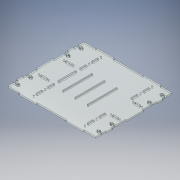
# Autodesk Inventor part: Base
Saved by Autodesk Inventor 2019 (Build 230136000, 136)
## iProperties
Created: 2020-04-02
Part Number: Base
Material: Acetal Resin, White
Document SubType Name: Modeling
Designer: Jurgen
Density: 1.425 g/cm^3
Appearance: Clear
Author: Jurgen
Autodesk Inventor part; units mm, degrees
(part 1 of 2)
ref_plane "YZ Plane" through (0, 0, 0) normal (1, 0, 0) x (0, 1, 0)
ref_plane "XZ Plane" through (0, 0, 0) normal (0, 1, 0) x (-1, 0, 0)
ref_plane "XY Plane" through (0, 0, 0) normal (0, 0, 1) x (1, 0, 0)
sketch "Sketch1" plane through (0, 0, 0) normal (0, 1, 0) x (-1, 0, 0)
  line L0 (-230, -200) -> (50, -200)
  line L1 (50, -200) -> (50, 60)
  line L2 (50, 60) -> (-230, 60)
  line L3 (-230, 60) -> (-230, -200)
  line L4 (-230, -200) -> (50, 60) construction
  line L5 (50, -200) -> (-230, 60) construction
  line L6 (0, 60) -> (0, -200) construction
  line L7 (-170, 60) -> (-170, -200) construction
  line L8 (50, -70) -> (-230, -70) construction
  line L9 (-90, 60) -> (-90, -200) construction
  dimension "d7" = 280
  dimension "d8" = 260
  dimension "d11" = 170
  dimension "d12" = 50
  constraints: 20 end point, 4 midpoint, 4 point on line, 2 horizontal, 2 parallel, 2 perpendicular, 1 vertical
  measures "d7" distance of L2.end L1.end
  measures "d8" distance of L1.end L0.end
  measures "d11" distance between parallel lines of L7 L6
  measures "d12" distance between parallel lines of L1 L6
extrude "Extrusion2" add sketch "Sketch1" along normal blind 5
sketch "Sketch2" plane through (0, 5, 0) normal (0, 1, 0) x (1, 0, 0)
  line L0 (230, 200) -> (-50, 200) construction
  line L1 (-50, 200) -> (-50, -60) construction
  line L2 (-50, -60) -> (230, -60) construction
  line L3 (230, -60) -> (230, 200) construction
  line L4 (-50, -60) -> (230, -60) construction
  line L5 (0, -60) -> (0, 200) construction
  line L6 (180, -60) -> (180, 200) construction
  line L7 (0, -35) -> (5, -35)
  line L8 (5, -35) -> (5, 25)
  line L9 (5, 25) -> (0, 25)
  line L10 (0, 25) -> (0, -35)
  line L11 (0, 115) -> (5, 115)
  line L12 (5, 115) -> (5, 175)
  line L13 (5, 175) -> (0, 175)
  line L14 (0, 175) -> (0, 115)
  line L15 (180, -35) -> (175, -35)
  line L16 (175, -35) -> (175, 25)
  line L17 (175, 25) -> (180, 25)
  line L18 (180, 25) -> (180, -35)
  line L19 (180, 115) -> (175, 115)
  line L20 (175, 115) -> (175, 175)
  line L21 (175, 175) -> (180, 175)
  line L22 (180, 175) -> (180, 115)
  point P0 (0, 0)
  dimension "d24" = 180
  dimension "d25" = 50
  dimension "d26" = 5
  dimension "d27" = 60
  dimension "d28" = 25
  dimension "d29" = 5
  dimension "d30" = 60
  dimension "d31" = 25
  dimension "d32" = 5
  dimension "d33" = 60
  dimension "d34" = 5
  dimension "d35" = 60
  dimension "d36" = 25
  dimension "d37" = 25
  constraints: 36 end point, 8 parallel, 8 point on line, 6 perpendicular, 4 horizontal
  measures "d24" distance between parallel lines of L6 L5
  measures "d25" distance between parallel lines of L1 L5
  measures "d26" distance of L9.end L8.end
  measures "d27" distance of L8.end L7.end
  measures "d28" distance between parallel lines of L2 L7
  measures "d29" distance of L13.end L12.end
  measures "d30" distance of L12.end L11.end
  measures "d31" distance between parallel lines of L0 L13
  measures "d32" distance of L16.end L17.end
  measures "d33" distance of L15.end L16.end
  measures "d34" distance of L20.end L21.end
  measures "d35" distance of L19.end L20.end
  measures "d36" distance from line of L2 L15.end
  measures "d37" distance from line of L6.end L21
extrude "Extrusion3" cut sketch "Sketch2" against normal blind 5
sketch "Sketch3" plane through (0, 5, 0) normal (0, 1, 0) x (1, 0, 0)
  line L0 (180, 25) -> (180, -35) construction
  line L1 (180, -35) -> (175, -35) construction
  line L2 (175, -35) -> (175, 25) construction
  line L3 (175, 25) -> (180, 25) construction
  line L4 (5, 25) -> (5, -35) construction
  line L5 (5, -35) -> (0, -35) construction
  line L6 (0, -35) -> (0, 25) construction
  line L7 (0, 25) -> (5, 25) construction
  line L8 (5, 175) -> (5, 115) construction
  line L9 (5, 115) -> (0, 115) construction
  line L10 (0, 115) -> (0, 175) construction
  line L11 (0, 175) -> (5, 175) construction
  line L12 (180, 175) -> (180, 115) construction
  line L13 (180, 115) -> (175, 115) construction
  line L14 (175, 115) -> (175, 175) construction
  line L15 (175, 175) -> (180, 175) construction
  line L16 (230, 200) -> (-50, 200) construction
  line L17 (-50, 200) -> (-50, -60) construction
  line L18 (-50, -60) -> (230, -60) construction
  line L19 (230, -60) -> (230, 200) construction
  line L20 (90, 200) -> (90, -60) construction
  line L21 (-50, -60) -> (230, -60) construction
  line L22 (-50, 200) -> (-50, -60) construction
  line L23 (-50, 70) -> (230, 70) construction
  line L24 (190, -60) -> (190, 200) construction
  line L25 (205, 30) -> (225, 30)
  line L26 (225, 30) -> (225, 25)
  line L27 (225, 25) -> (205, 25)
  line L28 (205, 25) -> (205, 30)
  line L29 (205, 110) -> (225, 110)
  line L30 (225, 110) -> (225, 115)
  line L31 (225, 115) -> (205, 115)
  line L32 (205, 115) -> (205, 110)
  line L33 (-25, 30) -> (-45, 30)
  line L34 (-45, 30) -> (-45, 25)
  line L35 (-45, 25) -> (-25, 25)
  line L36 (-25, 25) -> (-25, 30)
  line L37 (-45, 115) -> (-25, 115)
  line L38 (-45, 110) -> (-45, 115)
  line L39 (-25, 110) -> (-45, 110)
  line L40 (-25, 115) -> (-25, 110)
  point P0 (0, 0)
  dimension "d40" = 20
  dimension "d41" = 5
  dimension "d43" = 15
  dimension "d48" = 30
  dimension "d58" = 80
  constraints: 38 end point, 12 symmetric about line, 4 midpoint, 2 parallel, 2 perpendicular, 2 point on line, 1 horizontal
  measures "d40" distance of L26.end L27.end
  measures "d41" distance of L25.end L26.end
  measures "d43" distance between parallel lines of L24 L28
  measures "d48" distance from line of L29.start L14
  measures "d58" distance between parallel lines of L25 L29
extrude "Extrusion5" cut sketch "Sketch3" against normal blind 10 contours L36 L35 L34 L33 | L37 L40 L39 L38
sketch "Sketch6" plane through (0, 5, 0) normal (0, 1, 0) x (1, 0, 0)
  line L0 (-45, 115) -> (-25, 115) construction
  line L1 (-25, 115) -> (-25, 110) construction
  line L2 (-25, 110) -> (-45, 110) construction
  line L3 (-45, 30) -> (-25, 30) construction
  line L4 (-25, 30) -> (-25, 25) construction
  line L5 (-25, 25) -> (-45, 25) construction
  line L6 (180, 25) -> (180, -35) construction
  line L7 (180, -35) -> (175, -35) construction
  line L8 (175, -35) -> (175, 25) construction
  line L9 (175, 25) -> (180, 25) construction
  line L10 (5, 25) -> (5, -35) construction
  line L11 (5, -35) -> (0, -35) construction
  line L12 (0, -35) -> (0, 25) construction
  line L13 (0, 25) -> (5, 25) construction
  line L14 (5, 175) -> (5, 115) construction
  line L15 (5, 115) -> (0, 115) construction
  line L16 (0, 115) -> (0, 175) construction
  line L17 (0, 175) -> (5, 175) construction
  line L18 (180, 175) -> (180, 115) construction
  line L19 (180, 115) -> (175, 115) construction
  line L20 (175, 115) -> (175, 175) construction
  line L21 (175, 175) -> (180, 175) construction
  line L22 (230, 200) -> (-50, 200) construction
  line L23 (-50, 200) -> (-50, -60) construction
  line L24 (-50, -60) -> (230, -60) construction
  line L25 (230, -60) -> (230, 200) construction
  line L26 (230, 200) -> (-50, 200) projected
  line L27 (-50, -60) -> (230, -60) projected
  line L28 (230, 200) -> (210, 200)
  line L29 (210, 200) -> (210, -60)
  line L30 (210, -60) -> (230, -60)
  line L31 (230, -60) -> (230, 200)
  line L32 (-45, 110) -> (-45, 115) projected
  line L33 (-45, 25) -> (-45, 30) projected
  point P0 (0, 0)
  dimension "d51" = 20
  constraints: 8 end point, 2 parallel, 1 horizontal, 1 perpendicular, 1 point on line
  measures "d51" distance of L30.end L29.end
extrude "Extrusion7" cut sketch "Sketch6" against normal blind 10
sketch "Sketch7" plane through (0, 5, 0) normal (0, 1, 0) x (1, 0, 0)
  line L0 (210, -60) -> (210, 200) construction
  line L1 (210, 200) -> (-50, 200) construction
  line L2 (-50, 200) -> (-50, -60) construction
  line L3 (-50, -60) -> (210, -60) construction
  line L4 (180, 175) -> (180, 115) construction
  line L5 (180, 115) -> (175, 115) construction
  line L6 (175, 115) -> (175, 175) construction
  line L7 (175, 175) -> (180, 175) construction
  line L8 (5, 175) -> (5, 115) construction
  line L9 (5, 115) -> (0, 115) construction
  line L10 (0, 115) -> (0, 175) construction
  line L11 (0, 175) -> (5, 175) construction
  line L12 (5, 25) -> (5, -35) construction
  line L13 (5, -35) -> (0, -35) construction
  line L14 (0, -35) -> (0, 25) construction
  line L15 (0, 25) -> (5, 25) construction
  line L16 (180, 25) -> (180, -35) construction
  line L17 (180, -35) -> (175, -35) construction
  line L18 (175, -35) -> (175, 25) construction
  line L19 (175, 25) -> (180, 25) construction
  line L20 (-45, 30) -> (-25, 30) construction
  line L21 (-25, 30) -> (-25, 25) construction
  line L22 (-25, 25) -> (-45, 25) construction
  line L23 (-45, 115) -> (-25, 115) construction
  line L24 (-25, 115) -> (-25, 110) construction
  line L25 (-25, 110) -> (-45, 110) construction
  line L26 (-50, 200) -> (-70, 200)
  line L27 (-70, 200) -> (-70, -60)
  line L28 (-70, -60) -> (-50, -60)
  line L29 (-50, -60) -> (-50, 200)
  line L30 (-45, 25) -> (-45, 30) projected
  line L31 (-45, 110) -> (-45, 115) projected
  point P0 (0, 0)
  dimension "d54" = 20
  dimension "d57" = 260
  constraints: 8 end point, 2 parallel, 1 horizontal, 1 perpendicular
  measures "d54" distance of L28.end L27.end
  measures "d57" distance of L26.end L27.end
extrude "Extrusion8" add sketch "Sketch7" against normal blind 5
sketch "Sketch8" plane through (210, 5, 60) normal (1, 0, 0) x (0, 0, -1)
  line L0 (260, -5) -> (0, -5) projected
  line L1 (260, 0) -> (260, -5) projected
  line L2 (0, 0) -> (260, 0) projected
  line L3 (0, -5) -> (0, 0) projected
  point P0 (60, -5)
extrude "Extrusion9" add sketch "Sketch8" along normal blind 20
sketch "Sketch9" plane through (0, 5, 0) normal (0, 1, 0) x (1, 0, 0)
  line L0 (230, 200) -> (-70, 200) construction
  line L1 (-70, 200) -> (-70, -60) construction
  line L2 (-70, -60) -> (230, -60) construction
  line L3 (230, 200) -> (230, -60) construction
  line L4 (180, 175) -> (180, 115) construction
  line L5 (180, 115) -> (175, 115) construction
  line L6 (175, 115) -> (175, 175) construction
  line L7 (175, 175) -> (180, 175) construction
  line L8 (5, 175) -> (5, 115) construction
  line L9 (5, 115) -> (0, 115) construction
  line L10 (0, 115) -> (0, 175) construction
  line L11 (0, 175) -> (5, 175) construction
  line L12 (5, 25) -> (5, -35) construction
  line L13 (5, -35) -> (0, -35) construction
  line L14 (0, -35) -> (0, 25) construction
  line L15 (0, 25) -> (5, 25) construction
  line L16 (180, 25) -> (180, -35) construction
  line L17 (180, -35) -> (175, -35) construction
  line L18 (175, -35) -> (175, 25) construction
  line L19 (175, 25) -> (180, 25) construction
  line L20 (-45, 30) -> (-25, 30) construction
  line L21 (-25, 30) -> (-25, 25) construction
  line L22 (-25, 25) -> (-45, 25) construction
  line L23 (-45, 115) -> (-25, 115) construction
  line L24 (-25, 115) -> (-25, 110) construction
  line L25 (-25, 110) -> (-45, 110) construction
  line L26 (5, 115) -> (5, 135) construction
  line L27 (5, 175) -> (5, 115) construction
  line L28 (0, 115) -> (0, 175) construction
  line L29 (5, 135) -> (0, 135)
  line L30 (0, 135) -> (0, 155)
  line L31 (0, 155) -> (5, 155)
  line L32 (5, 155) -> (5, 135)
  line L33 (2.5, 155) -> (2.5, 135) construction
  line L34 (0, 145) -> (5, 145) construction
  circle A0 centre (2.5, 145) radius 2
  line L35 (5, 115) -> (0, 115) construction
  line L36 (2.5, 115) -> (2.5, 200) construction
  line L37 (230, 200) -> (-70, 200) construction
  circle A1 centre (2.5, 185) radius 2
  line L38 (180, 135) -> (175, 135)
  line L39 (175, 135) -> (175, 155)
  line L40 (175, 155) -> (180, 155)
  line L41 (180, 155) -> (180, 135)
  line L42 (177.5, 155) -> (177.5, 135) construction
  line L43 (175, 145) -> (180, 145) construction
  circle A2 centre (177.5, 145) radius 2
  circle A3 centre (177.5, 185) radius 2
  line L44 (5, -15) -> (0, -15)
  line L45 (0, -15) -> (0, 5)
  line L46 (0, 5) -> (5, 5)
  line L47 (5, 5) -> (5, -15)
  line L48 (2.5, 5) -> (2.5, -15) construction
  line L49 (0, -5) -> (5, -5) construction
  circle A4 centre (2.5, -5) radius 2
  circle A5 centre (2.5, 35) radius 2
  line L50 (180, -15) -> (175, -15)
  line L51 (175, -15) -> (175, 5)
  line L52 (175, 5) -> (180, 5)
  line L53 (180, 5) -> (180, -15)
  line L54 (177.5, 5) -> (177.5, -15) construction
  line L55 (175, -5) -> (180, -5) construction
  circle A6 centre (177.5, -5) radius 2
  circle A7 centre (177.5, 35) radius 2
  line L56 (-45, 25) -> (-45, 30) projected
  line L57 (-45, 110) -> (-45, 115) projected
  point P0 (0, 0)
  dimension "d61" = 20
  dimension "d65" = 20
  dimension "d66" = 4
  dimension "d67" = 4
  dimension "d68" = 10
  dimension "d69" = 20
  dimension "d70" = 4
  dimension "d71" = 4
  dimension "d72" = 20
  dimension "d73" = 4
  dimension "d74" = 4
  dimension "d75" = 20
  dimension "d76" = 4
  dimension "d77" = 4
  constraints: 52 end point, 21 midpoint, 8 centre point, 8 parallel, 5 perpendicular, 4 horizontal, 4 point on line
  measures "d61" distance of L8.end L26.end
  measures "d65" distance of L29.end L30.end
  measures "d66" diameter of A0
  measures "d67" diameter of A1
  measures "d68" distance from line of L11 A1.centre
  measures "d69" distance of L38.end L40.start
  measures "d70" diameter of A2
  measures "d71" diameter of A3
  measures "d72" distance of L44.end L46.start
  measures "d73" diameter of A4
  measures "d74" diameter of A5
  measures "d75" distance of L50.end L52.start
  measures "d76" diameter of A6
  measures "d77" diameter of A7
extrude "Extrusion10" add sketch "Sketch9" against normal blind 5 contours L29 L30 L31 L32 | L38 L39 L40 L41 | L44 L45 L46 L47 | L50 L51 L52 L53
sketch "Sketch10" plane through (0, 5, 0) normal (0, 1, 0) x (1, 0, 0)
  line L0 (230, 200) -> (-70, 200) construction
  line L1 (-70, 200) -> (-70, -60) construction
  line L2 (-70, -60) -> (230, -60) construction
  line L3 (230, 200) -> (230, -60) construction
  line L4 (180, 175) -> (180, 115) construction
  line L5 (180, 115) -> (175, 115) construction
  line L6 (175, 115) -> (175, 175) construction
  line L7 (175, 175) -> (180, 175) construction
  line L8 (5, 175) -> (5, 115) construction
  line L9 (5, 115) -> (0, 115) construction
  line L10 (0, 115) -> (0, 175) construction
  line L11 (0, 175) -> (5, 175) construction
  line L12 (5, 25) -> (5, -35) construction
  line L13 (5, -35) -> (0, -35) construction
  line L14 (0, -35) -> (0, 25) construction
  line L15 (0, 25) -> (5, 25) construction
  line L16 (180, 25) -> (180, -35) construction
  line L17 (180, -35) -> (175, -35) construction
  line L18 (175, -35) -> (175, 25) construction
  line L19 (175, 25) -> (180, 25) construction
  line L20 (-40, 25) -> (-40, 30) construction
  line L21 (-40, 30) -> (-15, 30) construction
  line L22 (-15, 30) -> (-15, 25) construction
  line L23 (-15, 25) -> (-40, 25) construction
  line L24 (-40, 110) -> (-40, 115) construction
  line L25 (-40, 115) -> (-15, 115) construction
  line L26 (-15, 115) -> (-15, 110) construction
  line L27 (-15, 110) -> (-40, 110) construction
  line L28 (5, 115) -> (5, 135) construction
  line L29 (5, 175) -> (5, 115) construction
  line L30 (0, 115) -> (0, 175) construction
  line L31 (5, 135) -> (0, 135)
  line L32 (0, 135) -> (0, 155)
  line L33 (0, 155) -> (5, 155)
  line L34 (5, 155) -> (5, 135)
  line L35 (2.5, 155) -> (2.5, 135) construction
  line L36 (0, 145) -> (5, 145) construction
  circle A0 centre (2.5, 145) radius 2
  line L37 (5, 115) -> (0, 115) construction
  line L38 (2.5, 115) -> (2.5, 200) construction
  line L39 (230, 200) -> (-70, 200) construction
  circle A1 centre (2.5, 185) radius 2
  circle A2 centre (177.5, 185) radius 2
  line L40 (175, 155) -> (180, 155)
  line L41 (175, 145) -> (180, 145) construction
  circle A3 centre (177.5, 145) radius 2
  line L42 (180, 135) -> (175, 135)
  line L43 (180, 155) -> (180, 135)
  line L44 (175, 135) -> (175, 155)
  line L45 (177.5, 155) -> (177.5, 135) construction
  circle A4 centre (2.5, 35) radius 2
  line L46 (0, 5) -> (5, 5)
  line L47 (0, -5) -> (5, -5) construction
  circle A5 centre (2.5, -5) radius 2
  line L48 (5, -15) -> (0, -15)
  line L49 (5, 5) -> (5, -15)
  line L50 (0, -15) -> (0, 5)
  line L51 (2.5, 5) -> (2.5, -15) construction
  circle A6 centre (177.5, 35) radius 2
  line L52 (175, 5) -> (180, 5)
  line L53 (175, -5) -> (180, -5) construction
  circle A7 centre (177.5, -5) radius 2
  line L54 (180, -15) -> (175, -15)
  line L55 (180, 5) -> (180, -15)
  line L56 (175, -15) -> (175, 5)
  line L57 (177.5, 5) -> (177.5, -15) construction
  line L58 (-70, 200) -> (-70, -60) construction
  line L59 (-70, 70) -> (230, 70) construction
  line L60 (230, -60) -> (230, 200) construction
  line L61 (175, -35) -> (180, -35) construction
  line L62 (0, -35) -> (5, -35) construction
  circle A8 centre (2.5, -45) radius 2
  circle A9 centre (177.5, -45) radius 2
  point P0 (0, 0)
  point P1 (0, 0)
  dimension "d80" = 20
  dimension "d81" = 20
  dimension "d82" = 4
  dimension "d83" = 4
  dimension "d84" = 10
  dimension "d85" = 20
  dimension "d86" = 4
  dimension "d87" = 4
  dimension "d88" = 20
  dimension "d89" = 4
  dimension "d90" = 4
  dimension "d91" = 20
  dimension "d92" = 4
  dimension "d93" = 4
  constraints: 122 end point, 23 midpoint, 10 centre point, 8 parallel, 5 perpendicular, 4 horizontal, 4 point on line, 2 symmetric about line, 2 other
  measures "d80" distance of L8.end L28.end
  measures "d81" distance of L31.end L32.end
  measures "d82" diameter of A0
  measures "d83" diameter of A1
  measures "d84" distance from line of L11 A1.centre
  measures "d85" distance of L42.end L40.start
  measures "d86" diameter of A3
  measures "d87" diameter of A2
  measures "d88" distance of L48.end L46.start
  measures "d89" diameter of A5
  measures "d90" diameter of A4
  measures "d91" distance of L54.end L52.start
  measures "d92" diameter of A7
  measures "d93" diameter of A6
extrude "Extrusion11" cut sketch "Sketch10" against normal blind 5 contours A1 | A2 | A8 | A9
sketch "Sketch11" plane through (0, 5, 0) normal (0, 1, 0) x (1, 0, 0)
  circle A0 centre (177.5, -45) radius 2 construction
  circle A1 centre (2.5, 185) radius 2 construction
  circle A2 centre (177.5, 185) radius 2 construction
  circle A3 centre (2.5, -45) radius 2 construction
  line L0 (0, 5) -> (0, 25) construction
  line L1 (0, 25) -> (5, 25) construction
  line L2 (5, 25) -> (5, 5) construction
  line L3 (5, 5) -> (0, 5) construction
  circle A4 centre (2.5, -5) radius 2 construction
  line L4 (5, 135) -> (5, 115) construction
  line L5 (5, 115) -> (0, 115) construction
  line L6 (0, 115) -> (0, 135) construction
  line L7 (5, 135) -> (0, 135) construction
  circle A5 centre (2.5, 145) radius 2 construction
  line L8 (175, 155) -> (175, 175) construction
  line L9 (175, 175) -> (180, 175) construction
  line L10 (180, 175) -> (180, 155) construction
  line L11 (180, 155) -> (175, 155) construction
  circle A6 centre (177.5, 145) radius 2 construction
  line L12 (175, 5) -> (175, 25) construction
  line L13 (175, 25) -> (180, 25) construction
  line L14 (180, 25) -> (180, 5) construction
  line L15 (180, 5) -> (175, 5) construction
  circle A7 centre (177.5, -5) radius 2 construction
  line L16 (230, 200) -> (-70, 200) construction
  line L17 (-70, 200) -> (-70, -60) construction
  line L18 (-70, -60) -> (230, -60) construction
  line L19 (230, 200) -> (230, -60) construction
  line L20 (175, 135) -> (180, 135) construction
  line L21 (180, 135) -> (180, 115) construction
  line L22 (180, 115) -> (175, 115) construction
  line L23 (175, 115) -> (175, 135) construction
  line L24 (0, 155) -> (5, 155) construction
  line L25 (0, 155) -> (0, 175) construction
  line L26 (0, 175) -> (5, 175) construction
  line L27 (5, 175) -> (5, 155) construction
  line L28 (0, -15) -> (5, -15) construction
  line L29 (5, -15) -> (5, -35) construction
  line L30 (5, -35) -> (0, -35) construction
  line L31 (0, -35) -> (0, -15) construction
  line L32 (175, -15) -> (180, -15) construction
  line L33 (180, -15) -> (180, -35) construction
  line L34 (180, -35) -> (175, -35) construction
  line L35 (175, -35) -> (175, -15) construction
  line L36 (-45, 25) -> (-45, 30) construction
  line L37 (-45, 30) -> (-25, 30) construction
  line L38 (-25, 30) -> (-25, 25) construction
  line L39 (-25, 25) -> (-45, 25) construction
  line L40 (-45, 110) -> (-45, 115) construction
  line L41 (-45, 115) -> (-25, 115) construction
  line L42 (-25, 115) -> (-25, 110) construction
  line L43 (-25, 110) -> (-45, 110) construction
  line L44 (-70, -60) -> (-70, 200) construction
  line L45 (-70, 112.5) -> (0, 112.5) construction
  line L46 (-70, 27.5) -> (0, 27.5) construction
  circle A8 centre (-51, 112.5) radius 2
  circle A9 centre (-19, 112.5) radius 2
  line L47 (-70, 70) -> (10.9855, 70) construction
  circle A10 centre (-51, 27.5) radius 2
  circle A11 centre (-19, 27.5) radius 2
  point P0 (0, 0)
  dimension "d96" = 4
  dimension "d97" = 6
  dimension "d98" = 4
  dimension "d99" = 6
  constraints: 6 end point, 4 centre point, 4 point on line, 2 horizontal, 2 symmetric about line, 1 midpoint, 1 perpendicular, 2 other
  measures "d96" diameter of A8
  measures "d97" distance from line of L40 A8.centre
  measures "d98" diameter of A9
  measures "d99" distance from line of L42 A9.centre
extrude "Extrusion12" cut sketch "Sketch11" against normal blind 10
sketch "Sketch12" plane through (0, 5, 0) normal (0, 1, 0) x (1, 0, 0)
  line L0 (196, 30) -> (214, 30)
  line L1 (214, 30) -> (214, 35)
  line L2 (214, 35) -> (196, 35)
  line L3 (196, 35) -> (196, 30)
  line L4 (196, 30) -> (214, 35) construction
  line L5 (214, 30) -> (196, 35) construction
  line L6 (-70, -60) -> (230, -60) construction
  line L7 (230, 200) -> (230, -60) construction
  line L8 (196, 32.5) -> (214, 32.5) construction
  line L9 (196, 32.5) -> (180, 32.5) construction
  line L10 (180, 32.5) -> (230, 32.5) construction
  circle A0 centre (220, 32.5) radius 2
  circle A1 centre (190, 32.5) radius 2
  line L11 (230, 70) -> (80, 70) construction
  line L12 (196, 110) -> (214, 110)
  line L13 (214, 110) -> (214, 105)
  line L14 (214, 105) -> (196, 105)
  line L15 (196, 105) -> (196, 110)
  line L16 (196, 110) -> (214, 105) construction
  line L17 (214, 110) -> (196, 105) construction
  line L18 (196, 107.5) -> (214, 107.5) construction
  line L19 (196, 107.5) -> (180, 107.5) construction
  circle A2 centre (220, 107.5) radius 2
  circle A3 centre (190, 107.5) radius 2
  point P0 (0, 0)
  point P1 (205, 32.5)
  point P2 (205, 107.5)
  dimension "d102" = 18
  dimension "d103" = 5
  dimension "d104" = 90
  dimension "d105" = 16
  dimension "d106" = 16
  dimension "d107" = 4
  dimension "d108" = 4
  dimension "d109" = 6
  dimension "d110" = 6
  constraints: 36 end point, 10 symmetric about line, 7 midpoint, 6 point on line, 4 centre point, 2 horizontal, 2 parallel, 1 perpendicular, 2 other
  measures "d102" distance of L2.end L1.end
  measures "d103" distance of L1.end L0.end
  measures "d104" distance between parallel lines of L6 L0
  measures "d105" distance between parallel lines of L7 L1
  measures "d106" distance of L8.start L9.end
  measures "d107" diameter of A0
  measures "d108" diameter of A1
  measures "d109" distance from line of L3 A1.centre
  measures "d110" distance from line of A0.centre L1
extrude "Extrusion13" cut sketch "Sketch12" against normal blind 10
sketch "Sketch13" plane through (0, 5, 0) normal (0, 1, 0) x (1, 0, 0)
  line L0 (214, 35) -> (214, 30) construction
  line L1 (214, 30) -> (196, 30) construction
  line L2 (196, 30) -> (196, 35) construction
  line L3 (196, 35) -> (214, 35) construction
  circle A0 centre (190, 107.5) radius 2 construction
  circle A1 centre (220, 32.5) radius 2 construction
  circle A2 centre (190, 32.5) radius 2 construction
  circle A3 centre (220, 107.5) radius 2 construction
  line L4 (196, 110) -> (214, 110) construction
  line L5 (214, 110) -> (214, 105) construction
  line L6 (214, 105) -> (196, 105) construction
  line L7 (196, 105) -> (196, 110) construction
  circle A4 centre (-51, 27.5) radius 2 construction
  circle A5 centre (-51, 112.5) radius 2 construction
  circle A6 centre (-19, 112.5) radius 2 construction
  circle A7 centre (-19, 27.5) radius 2 construction
  circle A8 centre (177.5, -45) radius 2 construction
  circle A9 centre (2.5, 185) radius 2 construction
  circle A10 centre (177.5, 185) radius 2 construction
  circle A11 centre (2.5, -45) radius 2 construction
  line L8 (0, 5) -> (0, 25) construction
  line L9 (0, 25) -> (5, 25) construction
  line L10 (5, 25) -> (5, 5) construction
  line L11 (5, 5) -> (0, 5) construction
  circle A12 centre (2.5, -5) radius 2 construction
  line L12 (5, 135) -> (5, 115) construction
  line L13 (5, 115) -> (0, 115) construction
  line L14 (0, 115) -> (0, 135) construction
  line L15 (5, 135) -> (0, 135) construction
  circle A13 centre (2.5, 145) radius 2 construction
  line L16 (175, 155) -> (175, 175) construction
  line L17 (175, 175) -> (180, 175) construction
  line L18 (180, 175) -> (180, 155) construction
  line L19 (180, 155) -> (175, 155) construction
  circle A14 centre (177.5, 145) radius 2 construction
  line L20 (175, 5) -> (175, 25) construction
  line L21 (175, 25) -> (180, 25) construction
  line L22 (180, 25) -> (180, 5) construction
  line L23 (180, 5) -> (175, 5) construction
  circle A15 centre (177.5, -5) radius 2 construction
  line L24 (230, 200) -> (-70, 200) construction
  line L25 (-70, 200) -> (-70, -60) construction
  line L26 (-70, -60) -> (230, -60) construction
  line L27 (230, 200) -> (230, -60) construction
  line L28 (175, 135) -> (180, 135) construction
  line L29 (180, 135) -> (180, 115) construction
  line L30 (180, 115) -> (175, 115) construction
  line L31 (175, 115) -> (175, 135) construction
  line L32 (0, 155) -> (5, 155) construction
  line L33 (0, 155) -> (0, 175) construction
  line L34 (0, 175) -> (5, 175) construction
  line L35 (5, 175) -> (5, 155) construction
  line L36 (0, -15) -> (5, -15) construction
  line L37 (5, -15) -> (5, -35) construction
  line L38 (5, -35) -> (0, -35) construction
  line L39 (0, -35) -> (0, -15) construction
  line L40 (175, -15) -> (180, -15) construction
  line L41 (180, -15) -> (180, -35) construction
  line L42 (180, -35) -> (175, -35) construction
  line L43 (175, -35) -> (175, -15) construction
  line L44 (-45, 25) -> (-45, 30) construction
  line L45 (-45, 30) -> (-25, 30) construction
  line L46 (-25, 30) -> (-25, 25) construction
  line L47 (-25, 25) -> (-45, 25) construction
  line L48 (-45, 110) -> (-45, 115) construction
  line L49 (-45, 115) -> (-25, 115) construction
  line L50 (-25, 115) -> (-25, 110) construction
  line L51 (-25, 110) -> (-45, 110) construction
  line L52 (192.5, 105) -> (192.5, 110) construction
  line L53 (192.5, 110) -> (217.5, 110) construction
  line L54 (217.5, 110) -> (217.5, 105) construction
  line L55 (217.5, 105) -> (192.5, 105) construction
  line L56 (217.5, 30) -> (192.5, 30) construction
  line L57 (192.5, 30) -> (192.5, 35) construction
  line L58 (192.5, 35) -> (217.5, 35) construction
  line L59 (217.5, 35) -> (217.5, 30) construction
  circle A16 centre (200, 85) radius 2 construction
  circle A17 centre (200, 55) radius 2 construction
  line L60 (212.5, -25) -> (212.5, -30) construction
  line L61 (212.5, -30) -> (197.5, -30) construction
  line L62 (197.5, -30) -> (197.5, -25) construction
  line L63 (197.5, -25) -> (212.5, -25) construction
  circle A18 centre (189.5, -27.5) radius 2 construction
  circle A19 centre (189.5, 176.5) radius 2 construction
  circle A20 centre (220.5, 176.5) radius 2 construction
  circle A21 centre (220.5, -27.5) radius 2 construction
  line L64 (212.5, 174) -> (197.5, 174) construction
  line L65 (197.5, 174) -> (197.5, 179) construction
  line L66 (197.5, 179) -> (212.5, 179) construction
  line L67 (212.5, 179) -> (212.5, 174) construction
  line L68 (232, 200) -> (177, 200) construction
  line L69 (177, 200) -> (177, 175) construction
  line L70 (177, 175) -> (182, 175) construction
  line L71 (182, 175) -> (182, 115) construction
  line L72 (182, 115) -> (177, 115) construction
  line L73 (177, 115) -> (177, 25) construction
  line L74 (177, 25) -> (182, 25) construction
  line L75 (182, 25) -> (182, -35) construction
  line L76 (182, -35) -> (177, -35) construction
  line L77 (177, -35) -> (177, -60) construction
  line L78 (177, -60) -> (232, -60) construction
  line L79 (232, -60) -> (232, -36) construction
  line L80 (232, -36) -> (235.5, -36) construction
  line L81 (235.5, -36) -> (235.5, -16) construction
  line L82 (235.5, -16) -> (232, -16) construction
  line L83 (232, -16) -> (232, 40) construction
  line L84 (232, 40) -> (235.5, 40) construction
  line L85 (235.5, 40) -> (235.5, 100) construction
  line L86 (235.5, 100) -> (232, 100) construction
  line L87 (232, 100) -> (232, 156) construction
  line L88 (235.5, 156) -> (232, 156) construction
  line L89 (232, 176) -> (235.5, 176) construction
  line L90 (232, 176) -> (232, 200) construction
  line L91 (205, 30) -> (205, 25) construction
  line L92 (205, 25) -> (185, 25) construction
  line L93 (185, 25) -> (185, 30) construction
  line L94 (185, 30) -> (205, 30) construction
  line L95 (205, 115) -> (205, 110) construction
  line L96 (205, 110) -> (185, 110) construction
  line L97 (185, 110) -> (185, 115) construction
  line L98 (185, 115) -> (205, 115) construction
  circle A22 centre (174.5, 167.5) radius 2 construction
  circle A23 centre (174.5, -36.5) radius 2 construction
  circle A24 centre (215.5, -36.5) radius 2 construction
  circle A25 centre (215.5, 167.5) radius 2 construction
  line L99 (182.5, 165) -> (182.5, 170) construction
  line L100 (182.5, 170) -> (207.5, 170) construction
  line L101 (207.5, 170) -> (207.5, 165) construction
  line L102 (207.5, 165) -> (182.5, 165) construction
  line L103 (207.5, -39) -> (182.5, -39) construction
  line L104 (182.5, -39) -> (182.5, -34) construction
  line L105 (182.5, -34) -> (207.5, -34) construction
  line L106 (207.5, -34) -> (207.5, -39) construction
  line L107 (157, -50) -> (230, -50) construction
  line L108 (230, -50) -> (230, -26) construction
  line L109 (230, -26) -> (235.5, -26) construction
  line L110 (235.5, -26) -> (235.5, -6) construction
  line L111 (235.5, -6) -> (232, -6) construction
  line L112 (232, -6) -> (232, 50) construction
  line L113 (232, 50) -> (235.5, 50) construction
  line L114 (235.5, 50) -> (235.5, 100) construction
  line L115 (235.5, 100) -> (230, 100) construction
  line L116 (230, 100) -> (230, 156) construction
  line L117 (233.5, 156) -> (230, 156) construction
  line L118 (233.5, 176) -> (233.5, 156) construction
  line L119 (232, 176) -> (233.5, 176) construction
  line L120 (232, 176) -> (232, 210) construction
  line L121 (232, 210) -> (157, 210) construction
  line L122 (157, 210) -> (157, 185) construction
  line L123 (157, 185) -> (162, 185) construction
  line L124 (162, 185) -> (162, 125) construction
  line L125 (162, 125) -> (157, 125) construction
  line L126 (157, 125) -> (157, 35) construction
  line L127 (157, 35) -> (162, 35) construction
  line L128 (162, 35) -> (162, -25) construction
  line L129 (162, -25) -> (157, -25) construction
  line L130 (157, -25) -> (157, -50) construction
  line L131 (230, -50) -> (230, -26) construction
  line L132 (230, -40) -> (213, -40) construction
  line L133 (213, -40) -> (213, -36) construction
  line L134 (213, -36) -> (230, -36) construction
  line L135 (230, -36) -> (230, -40) construction
  line L136 (213, -38) -> (230, -38) construction
  line L137 (221, -42) -> (217, -42) construction
  line L138 (217, -42) -> (217, -34) construction
  line L139 (217, -34) -> (221, -34) construction
  line L140 (221, -34) -> (221, -42) construction
  line L141 (221, -42) -> (217, -34) construction
  line L142 (217, -42) -> (221, -34) construction
  line L143 (230, -40) -> (221, -40)
  line L144 (221, -40) -> (221, -42)
  line L145 (221, -42) -> (217, -42)
  line L146 (217, -42) -> (217, -40)
  line L147 (217, -40) -> (213, -40)
  line L148 (213, -40) -> (213, -36)
  line L149 (213, -36) -> (217, -36)
  line L150 (217, -36) -> (217, -34)
  line L151 (217, -34) -> (221, -34)
  line L152 (221, -34) -> (221, -36)
  line L153 (221, -36) -> (230, -36)
  line L154 (230, -40) -> (230, -36)
  line L155 (221, 4) -> (221, 2)
  line L156 (221, 2) -> (217, 2)
  line L157 (217, 2) -> (217, 4)
  line L158 (221, 2) -> (217, 2) construction
  line L159 (221, 10) -> (221, 8)
  line L160 (230, 4) -> (221, 4)
  line L161 (217, 10) -> (221, 10) construction
  line L162 (217, 10) -> (221, 10)
  line L163 (217, 8) -> (217, 10)
  line L164 (221, 10) -> (221, 2) construction
  line L165 (217, 4) -> (213, 4)
  line L166 (217, 2) -> (221, 10) construction
  line L167 (217, 2) -> (217, 10) construction
  line L168 (221, 2) -> (217, 10) construction
  line L169 (213, 8) -> (217, 8)
  line L170 (213, 4) -> (213, 8)
  line L171 (230, 4) -> (213, 4) construction
  line L172 (213, 8) -> (230, 8) construction
  line L173 (213, 6) -> (230, 6) construction
  line L174 (221, 8) -> (230, 8)
  line L175 (230, 4) -> (230, 8)
  line L176 (230, 8) -> (230, 4) construction
  line L177 (213, 4) -> (213, 8) construction
  line L178 (221, 132) -> (221, 130)
  line L179 (221, 130) -> (217, 130)
  line L180 (217, 130) -> (217, 132)
  line L181 (221, 130) -> (217, 130) construction
  line L182 (221, 138) -> (221, 136)
  line L183 (230, 132) -> (221, 132)
  line L184 (217, 138) -> (221, 138) construction
  line L185 (217, 138) -> (221, 138)
  line L186 (217, 136) -> (217, 138)
  line L187 (221, 138) -> (221, 130) construction
  line L188 (217, 132) -> (213, 132)
  line L189 (217, 130) -> (221, 138) construction
  line L190 (217, 130) -> (217, 138) construction
  line L191 (221, 130) -> (217, 138) construction
  line L192 (213, 136) -> (217, 136)
  line L193 (213, 132) -> (213, 136)
  line L194 (230, 132) -> (213, 132) construction
  line L195 (213, 136) -> (230, 136) construction
  line L196 (213, 134) -> (230, 134) construction
  line L197 (221, 136) -> (230, 136)
  line L198 (230, 132) -> (230, 136)
  line L199 (230, 136) -> (230, 132) construction
  line L200 (213, 132) -> (213, 136) construction
  line L201 (221, 176) -> (221, 174)
  line L202 (221, 174) -> (217, 174)
  line L203 (217, 174) -> (217, 176)
  line L204 (221, 174) -> (217, 174) construction
  line L205 (221, 182) -> (221, 180)
  line L206 (230, 176) -> (221, 176)
  line L207 (217, 182) -> (221, 182) construction
  line L208 (217, 182) -> (221, 182)
  line L209 (217, 180) -> (217, 182)
  line L210 (221, 182) -> (221, 174) construction
  line L211 (217, 176) -> (213, 176)
  line L212 (217, 174) -> (221, 182) construction
  line L213 (217, 174) -> (217, 182) construction
  line L214 (221, 174) -> (217, 182) construction
  line L215 (213, 180) -> (217, 180)
  line L216 (213, 176) -> (213, 180)
  line L217 (230, 176) -> (213, 176) construction
  line L218 (213, 180) -> (230, 180) construction
  line L219 (213, 178) -> (230, 178) construction
  line L220 (221, 180) -> (230, 180)
  line L221 (230, 176) -> (230, 180)
  line L222 (230, 180) -> (230, 176) construction
  line L223 (213, 176) -> (213, 180) construction
  line L224 (80, 200) -> (80, -60) construction
  line L225 (230, -60) -> (-70, -60) construction
  line L226 (-54, 35) -> (-54, 30) construction
  circle A26 centre (-60, 32.5) radius 2 construction
  circle A27 centre (-60, 107.5) radius 2 construction
  line L227 (-54, 110) -> (-54, 105) construction
  line L228 (-57.5, 110) -> (-57.5, 105) construction
  line L229 (-57.5, 35) -> (-57.5, 30) construction
  line L230 (-52.5, -25) -> (-52.5, -30) construction
  circle A28 centre (-60.5, 176.5) radius 2 construction
  circle A29 centre (-60.5, -27.5) radius 2 construction
  line L231 (-52.5, 179) -> (-52.5, 174) construction
  line L232 (-72, -36) -> (-75.5, -36) construction
  line L233 (-75.5, -36) -> (-75.5, -16) construction
  line L234 (-75.5, -16) -> (-72, -16) construction
  line L235 (-72, -16) -> (-72, 40) construction
  line L236 (-72, 40) -> (-75.5, 40) construction
  line L237 (-75.5, 40) -> (-75.5, 100) construction
  line L238 (-75.5, 100) -> (-72, 100) construction
  line L239 (-72, 100) -> (-72, 156) construction
  line L240 (-75.5, 156) -> (-72, 156) construction
  line L241 (-72, 176) -> (-75.5, 176) construction
  circle A30 centre (-55.5, -36.5) radius 2 construction
  circle A31 centre (-55.5, 167.5) radius 2 construction
  line L242 (-70, -26) -> (-75.5, -26) construction
  line L243 (-75.5, -26) -> (-75.5, -6) construction
  line L244 (-75.5, -6) -> (-72, -6) construction
  line L245 (-72, -6) -> (-72, 50) construction
  line L246 (-72, 50) -> (-75.5, 50) construction
  line L247 (-75.5, 50) -> (-75.5, 100) construction
  line L248 (-75.5, 100) -> (-70, 100) construction
  line L249 (-70, 100) -> (-70, 156) construction
  line L250 (-73.5, 156) -> (-70, 156) construction
  line L251 (-73.5, 176) -> (-73.5, 156) construction
  line L252 (-72, 176) -> (-73.5, 176) construction
  line L253 (-70, -40) -> (-53, -40) construction
  line L254 (-53, -40) -> (-53, -36) construction
  line L255 (-53, -36) -> (-70, -36) construction
  line L256 (-70, -36) -> (-70, -40) construction
  line L257 (-53, -38) -> (-70, -38) construction
  line L258 (-61, -42) -> (-57, -42) construction
  line L259 (-57, -42) -> (-57, -34) construction
  line L260 (-57, -34) -> (-61, -34) construction
  line L261 (-61, -34) -> (-61, -42) construction
  line L262 (-61, -42) -> (-57, -34) construction
  line L263 (-57, -42) -> (-61, -34) construction
  line L264 (-70, -40) -> (-61, -40)
  line L265 (-61, -40) -> (-61, -42)
  line L266 (-61, -42) -> (-57, -42)
  line L267 (-57, -42) -> (-57, -40)
  line L268 (-57, -40) -> (-53, -40)
  line L269 (-53, -40) -> (-53, -36)
  line L270 (-53, -36) -> (-57, -36)
  line L271 (-57, -36) -> (-57, -34)
  line L272 (-57, -34) -> (-61, -34)
  line L273 (-61, -34) -> (-61, -36)
  line L274 (-61, -36) -> (-70, -36)
  line L275 (-70, -40) -> (-70, -36)
  line L276 (-61, 4) -> (-61, 2)
  line L277 (-61, 2) -> (-57, 2)
  line L278 (-57, 2) -> (-57, 4)
  line L279 (-61, 2) -> (-57, 2) construction
  line L280 (-61, 10) -> (-61, 8)
  line L281 (-70, 4) -> (-61, 4)
  line L282 (-57, 10) -> (-61, 10) construction
  line L283 (-57, 10) -> (-61, 10)
  line L284 (-57, 8) -> (-57, 10)
  line L285 (-61, 10) -> (-61, 2) construction
  line L286 (-57, 4) -> (-53, 4)
  line L287 (-57, 2) -> (-61, 10) construction
  line L288 (-57, 2) -> (-57, 10) construction
  line L289 (-61, 2) -> (-57, 10) construction
  line L290 (-53, 8) -> (-57, 8)
  line L291 (-53, 4) -> (-53, 8)
  line L292 (-70, 4) -> (-53, 4) construction
  line L293 (-53, 8) -> (-70, 8) construction
  line L294 (-53, 6) -> (-70, 6) construction
  line L295 (-61, 8) -> (-70, 8)
  line L296 (-70, 4) -> (-70, 8)
  line L297 (-70, 8) -> (-70, 4) construction
  line L298 (-53, 4) -> (-53, 8) construction
  line L299 (-61, 132) -> (-61, 130)
  line L300 (-61, 130) -> (-57, 130)
  line L301 (-57, 130) -> (-57, 132)
  line L302 (-61, 130) -> (-57, 130) construction
  line L303 (-61, 138) -> (-61, 136)
  line L304 (-70, 132) -> (-61, 132)
  line L305 (-57, 138) -> (-61, 138) construction
  line L306 (-57, 138) -> (-61, 138)
  line L307 (-57, 136) -> (-57, 138)
  line L308 (-61, 138) -> (-61, 130) construction
  line L309 (-57, 132) -> (-53, 132)
  line L310 (-57, 130) -> (-61, 138) construction
  line L311 (-57, 130) -> (-57, 138) construction
  line L312 (-61, 130) -> (-57, 138) construction
  line L313 (-53, 136) -> (-57, 136)
  line L314 (-53, 132) -> (-53, 136)
  line L315 (-70, 132) -> (-53, 132) construction
  line L316 (-53, 136) -> (-70, 136) construction
  line L317 (-53, 134) -> (-70, 134) construction
  line L318 (-61, 136) -> (-70, 136)
  line L319 (-70, 132) -> (-70, 136)
  line L320 (-70, 136) -> (-70, 132) construction
  line L321 (-53, 132) -> (-53, 136) construction
  line L322 (-61, 176) -> (-61, 174)
  line L323 (-61, 174) -> (-57, 174)
  line L324 (-57, 174) -> (-57, 176)
  line L325 (-61, 174) -> (-57, 174) construction
  line L326 (-61, 182) -> (-61, 180)
  line L327 (-70, 176) -> (-61, 176)
  line L328 (-57, 182) -> (-61, 182) construction
  line L329 (-57, 182) -> (-61, 182)
  line L330 (-57, 180) -> (-57, 182)
  line L331 (-61, 182) -> (-61, 174) construction
  line L332 (-57, 176) -> (-53, 176)
  line L333 (-57, 174) -> (-61, 182) construction
  line L334 (-57, 174) -> (-57, 182) construction
  line L335 (-61, 174) -> (-57, 182) construction
  line L336 (-53, 180) -> (-57, 180)
  line L337 (-53, 176) -> (-53, 180)
  line L338 (-70, 176) -> (-53, 176) construction
  line L339 (-53, 180) -> (-70, 180) construction
  line L340 (-53, 178) -> (-70, 178) construction
  line L341 (-61, 180) -> (-70, 180)
  line L342 (-70, 176) -> (-70, 180)
  line L343 (-70, 180) -> (-70, 176) construction
  line L344 (-53, 176) -> (-53, 180) construction
  point P0 (0, 0)
  point P1 (205, 70)
  point P2 (219, -38)
  point P3 (219, 6)
  point P4 (219, 134)
  point P5 (219, 178)
  point P6 (-59, -38)
  point P7 (-59, 6)
  point P8 (-59, 134)
  point P9 (-59, 178)
  dimension "d113" = 17
  dimension "d114" = 4
  dimension "d115" = 4
  dimension "d116" = 8
  dimension "d118" = 17
  dimension "d119" = 4
  dimension "d120" = 4
  dimension "d121" = 8
  dimension "d122" = 17
  dimension "d123" = 4
  dimension "d124" = 4
  dimension "d125" = 8
  dimension "d126" = 17
  dimension "d127" = 4
  dimension "d128" = 4
  dimension "d129" = 8
  dimension "d133" = 20
  dimension "d134" = 40
  dimension "d135" = 20
  dimension "d136" = 40
  dimension "d161" = 0
  dimension "d162" = 4
  dimension "d163" = 0
  dimension "d164" = 0
  dimension "d165" = 4
  dimension "d166" = 0
  dimension "d167" = 0
  dimension "d168" = 4
  dimension "d169" = 0
  dimension "d170" = 4
  constraints: 584 end point, 110 symmetric about line, 81 point on line, 28 perpendicular, 26 midpoint, 16 centre point, 16 parallel, 8 collinear, 8 horizontal, 6 other
  measures "d113" distance of L133.end L134.end
  measures "d114" distance of L132.end L133.end
  measures "d115" distance of L138.end L139.end
  measures "d116" distance of L137.end L138.end
  measures "d118" distance of L169.start L172.end
  measures "d119" distance of L165.end L169.start
  measures "d120" distance of L161.start L159.start
  measures "d121" distance of L156.end L161.start
  measures "d122" distance of L192.start L195.end
  measures "d123" distance of L188.end L192.start
  measures "d124" distance of L184.start L182.start
  measures "d125" distance of L179.end L184.start
  measures "d126" distance of L215.start L218.end
  measures "d127" distance of L211.end L215.start
  measures "d128" distance of L207.start L205.start
  measures "d129" distance of L202.end L207.start
  measures "d133" distance between parallel lines of L143 L26
  measures "d134" distance between parallel lines of L153 L160
  measures "d135" distance between parallel lines of L220 L24
  measures "d136" distance between parallel lines of L206 L197
  measures "d161" distance between parallel lines of L27 L108
  measures "d162" distance between parallel lines of L148 L150
  measures "d163" distance between parallel lines of L83 L112
  measures "d164" distance between parallel lines of L27 L175
  measures "d165" distance between parallel lines of L177 L163
  measures "d166" distance between parallel lines of L116 L27
  measures "d167" distance between parallel lines of L116 L198
  measures "d168" distance between parallel lines of L193 L190
  measures "d169" distance between parallel lines of L27 L221
  measures "d170" distance between parallel lines of L216 L203
extrude "Extrusion14" cut sketch "Sketch13" against normal blind 10